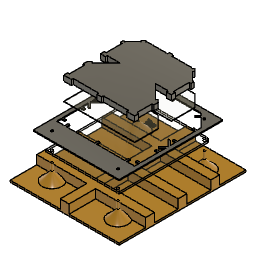
External Panels v20 (Autodesk Fusion 360 design; units mm, degrees)
Autodesk Fusion 360 part; units mm, degrees
note: some values were not read from the file. Chosen so that the rebuilt part matches the saved one: which bodies a step acts on; the layout of a text.
sketch "PCB" plane through (0, 0, 0) normal (0, 0, 1) x (1, 0, 0) in component "ExPan"
  line L0 (-41.5, 51.5) -> (38, 51.5)
  line L1 (41.5, 48) -> (41.5, -51.5)
  line L2 (41.5, -51.5) -> (-41.5, -51.5)
  line L3 (-41.5, -51.5) -> (-41.5, 51.5)
  line L4 (-41.5, 51.5) -> (41.5, -51.5) construction
  line L5 (41.5, 51.5) -> (-41.5, -51.5) construction
  circle A0 centre (-37.3, 49) radius 1.35
  line L6 (-41.5, 0) -> (41.5, 0) construction
  line L7 (0, 51.5) -> (0, -51.5) construction
  circle A1 centre (37.3, 49) radius 1.35
  circle A2 centre (-37.2, -48.5) radius 1.35
  circle A3 centre (37.2, -48.5) radius 1.35
  line L8 (38.907, 51.5) -> (38, 51.5) construction
  arc A4 (41.5, 48) -> (38, 51.5) centre (38, 48) ccw
  dimension "d14" = 83
  dimension "d15" = 103
  dimension "d16" = 2.7
  dimension "d18" = 4.2
  dimension "d19" = 2.5
  dimension "d24" = 2.7
  dimension "d25" = 4.3
  dimension "d26" = 3
  dimension "d141" = 3.5
  constraint horizontal L0
  constraint perpendicular L0 L1
  constraint parallel L0 L2
  constraint parallel L1 L3
  constraint coincident L4 origin
  constraint coincident L5 origin
  constraint midpoint L3 L6.start
  constraint midpoint L2 L7.end
  constraint symmetric A0 L7 A1
  constraint symmetric L7 A2 A3
  constraint horizontal L8
  constraint coincident L0 L8.start
  constraint coincident L1 L6.end
  constraint coincident L5.start L1
  constraint tangent L8 A4
  constraint tangent L1 A4
  constraint coincident L0 L7.start
  measures "d14" distance of L1 L3
  measures "d15" distance of L0 L2
  measures "d16" diameter of A0
  measures "d18" distance of L3 A0.centre
  measures "d19" distance of L0 A0.centre
  measures "d24" diameter of A2
  measures "d25" distance of L3 A2.centre
  measures "d26" distance of L2 A2.centre
  measures "d141" radius of A4
sketch "Base" plane through (0, 0, 0) normal (0, 0, 1) x (1, 0, 0) in component "ExPan"
  line L0 (61.5, -71.5) -> (-61.5, -71.5)
  line L1 (-61.5, -71.5) -> (-61.5, 71.5)
  line L2 (-61.5, 71.5) -> (61.5, 71.5)
  line L3 (61.5, 71.5) -> (61.5, -71.5)
  line L4 (61.5, -71.5) -> (-61.5, 71.5) construction
  line L5 (-61.5, -71.5) -> (61.5, 71.5) construction
  line L6 (41.5, -51.5) -> (-41.5, -51.5)
  line L7 (41.5, 48) -> (41.5, -51.5)
  circle A0 centre (37.2, -48.5) radius 1.1
  line L8 (0, 51.5) -> (0, -51.5) construction
  circle A1 centre (-37.2, -48.5) radius 1.1
  line L9 (-41.5, 0) -> (41.5, 0) construction
  circle A2 centre (37.3, 49) radius 1.1
  line L10 (-41.5, 51.5) -> (38, 51.5)
  circle A3 centre (-37.3, 49) radius 1.1
  line L11 (-61.5, -31.5) -> (61.5, -31.5)
  line L12 (61.5, -31.5) -> (61.5, -41.5)
  line L13 (61.5, -41.5) -> (-61.5, -41.5)
  line L14 (-61.5, -41.5) -> (-61.5, -31.5)
  line L15 (-61.5, 42) -> (61.5, 42)
  line L16 (61.5, 42) -> (61.5, 32)
  line L17 (61.5, 32) -> (-61.5, 32)
  line L18 (-61.5, 32) -> (-61.5, 42)
  line L19 (-5, 71.5) -> (5, 71.5)
  line L20 (5, 71.5) -> (5, -71.5)
  line L21 (5, -71.5) -> (-5, -71.5)
  line L22 (-5, -71.5) -> (-5, 71.5)
  line L23 (-61.5, 5) -> (61.5, 5)
  line L24 (61.5, 5) -> (61.5, -5)
  line L25 (61.5, -5) -> (-61.5, -5)
  line L26 (-61.5, -5) -> (-61.5, 5)
  line L27 (-42.5017, 60.3845) -> (-15.0062, 60.3658) construction
  line L28 (-15.0062, 60.3658) -> (-15.0027, 65.4577) construction
  line L29 (-15.0027, 65.4577) -> (-42.4983, 65.4765) construction
  line L30 (-42.4983, 65.4765) -> (-42.5017, 60.3845) construction
  point P0 (-37.3, 49)
  point P1 (37.3, 49)
  dimension "d35" = 20
  dimension "d36" = 20
  dimension "d37" = 2.2
  dimension "d38" = 3
  dimension "d39" = 4.3
  dimension "d40" = 2.2
  dimension "d41" = 4.2
  dimension "d42" = 2.5
  dimension "d119" = 10
  dimension "d120" = 7
  dimension "d121" = 7
  dimension "d122" = 10
  dimension "d123" = 10
  dimension "d129" = 10
  dimension "d130" = 5
  dimension "d131" = 5
  dimension "d134" = 5
  dimension "d139" = 19
  text T0 "Top" font "Arial" height 5 align left top in box 27.4956 x 5.0919 at (-42.5017, 60.3845) x (1, -0.000682) y (0.000682, 1) spacing 1 kerned
  constraint horizontal L0
  constraint perpendicular L0 L1
  constraint parallel L0 L2
  constraint parallel L1 L3
  constraint coincident L4 origin
  constraint coincident L5 origin
  constraint symmetric A0 L8 A1
  constraint symmetric L8 A2 A3
  constraint horizontal L11
  constraint vertical L12
  constraint horizontal L13
  constraint vertical L14
  constraint coincident L1 L11.start
  constraint horizontal L15
  constraint vertical L16
  constraint horizontal L17
  constraint vertical L18
  constraint coincident L3 L16.end
  constraint coincident L1 L15.start
  constraint horizontal L19
  constraint vertical L20
  constraint horizontal L21
  constraint vertical L22
  constraint coincident L0 L20.end
  constraint coincident L2 L19.start
  constraint horizontal L23
  constraint vertical L24
  constraint horizontal L25
  constraint vertical L26
  constraint coincident L3 L24.end
  constraint coincident L1 L23.start
  measures "d35" distance of L0 L6
  measures "d36" distance of L3 L7
  measures "d37" diameter of A0
  measures "d38" distance of L6 A0.centre
  measures "d39" distance of L7 A0.centre
  measures "d40" diameter of A2
  measures "d41" distance of L7 P1
  measures "d42" distance of P1 L10
  measures "d119" distance of L11.start L13.end
  measures "d120" distance of A1.centre L13
  measures "d121" distance of P0 L15
  measures "d122" distance of L15 L17
  measures "d123" distance of L20 L22
  measures "d129" distance of L23 L25
  measures "d130" distance of origin L23
  measures "d131" distance of origin L22
sketch "SC" plane through (0, 0, 0) normal (0, 0, 1) x (1, 0, 0) in component "ExPan"
  line L0 (-40, 9) -> (40, 9)
  line L1 (40, 9) -> (40, 35.5)
  line L2 (26.5, 49) -> (-26.5, 49)
  line L3 (-40, 35.5) -> (-40, 9)
  line L4 (-41.5, -51.5) -> (-41.5, 51.5)
  line L5 (-41.5, 51.5) -> (38, 51.5)
  line L6 (-40, 35.5) -> (-26.5, 49)
  line L7 (0, 51.5) -> (0, -51.5)
  line L8 (40, 35.5) -> (26.5, 49)
  line L9 (-40, -32.5) -> (40, -32.5)
  line L10 (40, -32.5) -> (40, -6)
  line L11 (26.5, 7.5) -> (-26.5, 7.5)
  line L12 (-40, -6) -> (-26.5, 7.5)
  line L13 (-40, -6) -> (-40, -32.5)
  line L14 (40, -6) -> (26.5, 7.5)
  dimension "d43" = 80
  dimension "d45" = 1.5
  dimension "d47" = 2.5
  dimension "d48" = 13.5
  dimension "d49" = 13.5
  dimension "d190" = 40
  dimension "d191" = 80
  dimension "d192" = 13.5
  dimension "d193" = 13.5
  dimension "d194" = 40
  dimension "d195" = 1.5
  dimension "d196" = 1.5
  constraint vertical L1
  constraint horizontal L2
  constraint vertical L3
  constraint coincident L3.start L6.start
  constraint coincident L2.end L6.end
  constraint symmetric L3.start L7 L1.end
  constraint symmetric L2.end L7 L2.start
  constraint vertical L10
  constraint horizontal L11
  constraint vertical L13
  constraint coincident L12.start L13.start
  constraint coincident L11.end L12.end
  constraint symmetric L7 L11.end L11.start
  constraint symmetric L7 L12.start L10.end
  measures "d43" distance of L0.start L0.end
  measures "d45" distance of L3 L4
  measures "d47" distance of L2 L5
  measures "d48" distance of L2 L3.start
  measures "d49" distance of L3 L2.end
  measures "d190" distance of L0 L2
  measures "d191" distance of L9.start L9.end
  measures "d192" distance of L12.start L11
  measures "d193" distance of L11.end L13
  measures "d194" distance of L9 L11
  measures "d195" distance of L0 L11
  measures "d196" distance of L4 L13
sketch "Mask" plane through (0, 0, 0) normal (0, 0, 1) x (1, 0, 0) in component "ExPan"
  line L0 (-45, 58.5) -> (48.5, 58.5)
  line L1 (48.5, 58.5) -> (48.5, -58.5)
  line L2 (48.5, -58.5) -> (-48.5, -58.5)
  line L3 (-48.5, -58.5) -> (-48.5, 58.5)
  line L4 (-41.5, -51.5) -> (-41.5, 51.5)
  line L5 (41.5, -51.5) -> (-41.5, -51.5)
  circle A0 centre (-37.2, -48.5) radius 1.35
  circle A1 centre (-37.3, 49) radius 1.35
  line L6 (-48.5, 58.5) -> (-45, 58.5)
  line L7 (44, -36.5) -> (44, 38.5711)
  line L8 (44, 38.5711) -> (29.5711, 53)
  line L9 (29.5711, 53) -> (-29.5711, 53)
  line L10 (-44, 38.5711) -> (-44, -36.5)
  line L11 (17.1694, 53) -> (17.1971, 53)
  line L12 (17.1971, 50.5) -> (17.1694, 50.5)
  line L13 (-41.5, 51.5) -> (38, 51.5)
  line L14 (-44, -36.5) -> (44, -36.5)
  line L15 (-29.5711, 53) -> (-44, 38.5711)
  line L16 (-40, 35.5) -> (-26.5, 49)
  line L17 (40, 35.5) -> (26.5, 49)
  line L18 (-40, -32.5) -> (40, -32.5)
  line L19 (0, 51.5) -> (0, -51.5)
  circle A2 centre (37.2, -48.5) radius 1.35
  circle A3 centre (37.3, 49) radius 1.35
  line L20 (-40.1, -6) -> (-40.1, -35)
  line L21 (-40, -6) -> (-40, -32.5)
  line L22 (-44, -31.4682) -> (-40.1, -31.4682)
  line L23 (-44, -29.4682) -> (-40.1, -29.4682)
  line L24 (40.1, -6) -> (40.1, -35)
  line L25 (-26.5404, 7.601) -> (-41.5185, -7.3771)
  line L26 (-26.5404, 7.601) -> (-5.482, 7.601) construction
  line L27 (-40, -6) -> (-26.5, 7.5)
  line L28 (-39.6133, -5.4719) -> (-44, -1.0852)
  line L29 (-39.6133, -5.4719) -> (-31.8598, -5.4719) construction
  line L30 (-38.1991, -4.0577) -> (-44, 1.7432)
  line L31 (-38.1991, -4.0577) -> (-31.6288, -4.0577) construction
  line L32 (-44, -7.8862) -> (-40.1, -7.8862)
  line L33 (-44, -9.8862) -> (-40.1, -9.8862)
  line L34 (-41, -32.6) -> (42, -32.6)
  line L35 (-34.94, -36.5) -> (-34.94, -32.6)
  line L36 (-32.94, -36.5) -> (-32.94, -32.6)
  line L37 (-1, -36.5) -> (-1, -32.6)
  line L38 (1, -36.5) -> (1, -32.6)
  line L39 (34.94, -36.5) -> (34.94, -32.6)
  line L40 (32.94, -36.5) -> (32.94, -32.6)
  line L41 (44, -31.4682) -> (40.1, -31.4682)
  line L42 (44, -29.4682) -> (40.1, -29.4682)
  line L43 (44, -9.8862) -> (40.1, -9.8862)
  line L44 (44, -7.8862) -> (40.1, -7.8862)
  line L45 (38.1991, -4.0577) -> (44, 1.7432)
  line L46 (39.6133, -5.4719) -> (44, -1.0852)
  line L47 (26.5404, 7.601) -> (41.5185, -7.3771)
  line L48 (26.5, 49) -> (-26.5, 49)
  line L49 (-26.1265, 49.15) -> (28.8735, 49.15)
  line L50 (-40.1, 8) -> (-40.1, 37)
  line L51 (-40, 35.5) -> (-40, 9)
  line L52 (-40.0495, 35.5919) -> (-25.6143, 50.0271)
  line L53 (-44, 34.0706) -> (-40.1, 34.0706)
  line L54 (-44, 32.0706) -> (-40.1, 32.0706)
  line L55 (-40.1, 11.9824) -> (-44, 11.9824)
  line L56 (-44, 9.9824) -> (-40.1, 9.9824)
  line L57 (-1, 53) -> (-1, 49.15)
  line L58 (-33.213, 49.358) -> (-29.7482, 45.8932)
  line L59 (-31.7988, 50.7723) -> (-28.334, 47.3074)
  line L60 (-41, 8.9) -> (42.4266, 8.9)
  line L61 (-40, 9) -> (40, 9)
  line L62 (39.1562, 8.9) -> (44, 4.0562)
  line L63 (39.1562, 8.9) -> (45.9442, 8.9) construction
  line L64 (36.3278, 8.9) -> (44.4159, 0.8118)
  line L65 (36.3278, 8.9) -> (47.7041, 8.9) construction
  line L66 (-36.3278, 8.9) -> (-44.4159, 0.8118)
  line L67 (-39.1562, 8.9) -> (-44, 4.0562)
  line L68 (33.213, 49.358) -> (29.7482, 45.8932)
  line L69 (31.7988, 50.7723) -> (28.334, 47.3074)
  line L70 (1, 53) -> (1, 49.15)
  line L71 (44, 34.0706) -> (40.1, 34.0706)
  line L72 (44, 32.0706) -> (40.1, 32.0706)
  line L73 (40.1, 11.9824) -> (44, 11.9824)
  line L74 (44, 9.9824) -> (40.1, 9.9824)
  line L75 (40.0495, 35.5919) -> (25.6143, 50.0271)
  line L76 (40.1, 8) -> (40.1, 37)
  dimension "d55" = 117
  dimension "d56" = 97
  dimension "d58" = 7
  dimension "d59" = 7
  dimension "d99" = 2.7
  dimension "d100" = 11.3
  dimension "d101" = 10
  dimension "d102" = 2.7
  dimension "d103" = 11.2
  dimension "d104" = 9.5
  dimension "d182" = 4.5
  dimension "d183" = 4.5
  dimension "d185" = 5
  dimension "d198" = 5
  dimension "d199" = 4
  dimension "d200" = 0.1
  dimension "d201" = 2
  dimension "d202" = 135
  dimension "d203" = 0.1
  dimension "d204" = 135
  dimension "d205" = 135
  dimension "d206" = 2
  dimension "d207" = 2
  dimension "d208" = 0.1
  dimension "d209" = 2
  dimension "d210" = 1
  dimension "d211" = 4
  dimension "d212" = 0.15
  dimension "d213" = 0.1
  dimension "d214" = 2
  dimension "d215" = 2
  dimension "d216" = 1
  dimension "d217" = 0.1
  dimension "d218" = 2
  dimension "d219" = 0.1
  dimension "d220" = 45
  dimension "d221" = 45
  dimension "d222" = 2
  constraint horizontal L0
  constraint vertical L1
  constraint horizontal L2
  constraint vertical L3
  constraint horizontal L6
  constraint vertical L10
  constraint horizontal L11
  constraint horizontal L12
  constraint coincident L9 L11.start
  constraint symmetric A0 L19 A2
  constraint symmetric A1 L19 A3
  constraint parallel L4 L20
  constraint coincident L10 L22.start
  constraint coincident L20 L22.end
  constraint perpendicular L20 L22
  constraint coincident L10 L23.start
  constraint coincident L20 L23.end
  constraint perpendicular L20 L23
  constraint symmetric L19 L20.start L24.start
  constraint symmetric L19 L20.end L24.end
  constraint horizontal L26
  constraint horizontal L29
  constraint coincident L25 L28.start
  constraint coincident L10 L28.end
  constraint horizontal L31
  constraint coincident L25 L30.start
  constraint coincident L10 L30.end
  constraint coincident L10 L32.start
  constraint coincident L20 L32.end
  constraint perpendicular L20 L32
  constraint coincident L10 L33.start
  constraint coincident L20 L33.end
  constraint perpendicular L20 L33
  constraint perpendicular L7 L34
  constraint coincident L14 L35.start
  constraint coincident L34 L35.end
  constraint perpendicular L34 L35
  constraint coincident L14 L36.start
  constraint coincident L34 L36.end
  constraint perpendicular L18 L36
  constraint coincident L14 L37.start
  constraint coincident L34 L37.end
  constraint perpendicular L34 L37
  constraint symmetric L19 L22.start L41.start
  constraint symmetric L19 L22.end L41.end
  constraint symmetric L19 L23.start L42.start
  constraint symmetric L19 L23.end L42.end
  constraint symmetric L19 L25.start L47.start
  constraint symmetric L19 L25.end L47.end
  constraint symmetric L19 L28.start L46.start
  constraint symmetric L19 L28.end L46.end
  constraint symmetric L19 L30.start L45.start
  constraint symmetric L19 L30.end L45.end
  constraint symmetric L19 L32.start L44.start
  constraint symmetric L19 L32.end L44.end
  constraint symmetric L19 L33.start L43.start
  constraint symmetric L19 L33.end L43.end
  constraint symmetric L19 L35.start L39.start
  constraint symmetric L19 L35.end L39.end
  constraint symmetric L19 L36.start L40.start
  constraint symmetric L19 L36.end L40.end
  constraint symmetric L19 L37.start L38.start
  constraint symmetric L19 L37.end L38.end
  constraint parallel L48 L49
  constraint parallel L4 L50
  constraint parallel L16 L52
  constraint coincident L10 L53.start
  constraint coincident L50 L53.end
  constraint perpendicular L50 L53
  constraint coincident L10 L54.start
  constraint coincident L50 L54.end
  constraint perpendicular L50 L54
  constraint coincident L50 L55.start
  constraint coincident L10 L55.end
  constraint perpendicular L10 L55
  constraint coincident L10 L56.start
  constraint coincident L50 L56.end
  constraint perpendicular L50 L56
  constraint coincident L9 L57.start
  constraint coincident L49 L57.end
  constraint perpendicular L49 L57
  constraint coincident L15 L58.start
  constraint coincident L52 L58.end
  constraint perpendicular L52 L58
  constraint coincident L15 L59.start
  constraint coincident L52 L59.end
  constraint perpendicular L52 L59
  constraint perpendicular L51 L60
  constraint horizontal L63
  constraint coincident L60 L62.start
  constraint coincident L7 L62.end
  constraint horizontal L65
  constraint coincident L60 L64.start
  constraint symmetric L19 L53.start L71.start
  constraint symmetric L19 L53.end L71.end
  constraint symmetric L19 L54.start L72.start
  constraint symmetric L19 L54.end L72.end
  constraint symmetric L19 L55.start L73.start
  constraint symmetric L19 L55.end L73.end
  constraint symmetric L19 L56.start L74.start
  constraint symmetric L19 L56.end L74.end
  constraint symmetric L19 L57.start L70.start
  constraint symmetric L19 L57.end L70.end
  constraint symmetric L19 L58.start L68.start
  constraint symmetric L19 L58.end L68.end
  constraint symmetric L19 L59.start L69.start
  constraint symmetric L19 L59.end L69.end
  constraint symmetric L19 L62.start L67.start
  constraint symmetric L19 L62.end L67.end
  constraint symmetric L19 L64.start L66.start
  constraint symmetric L19 L64.end L66.end
  constraint symmetric L19 L50.start L76.start
  constraint symmetric L19 L50.end L76.end
  constraint symmetric L19 L52.start L75.start
  constraint symmetric L19 L52.end L75.end
  measures "d55" distance of L0 L2
  measures "d56" distance of L1 L3
  measures "d58" distance of L3 L4
  measures "d59" distance of L2 L5
  measures "d99" diameter of A0
  measures "d100" distance of L3 A0.centre
  measures "d101" distance of L2 A0.centre
  measures "d102" diameter of A1
  measures "d103" distance of L3 A1.centre
  measures "d104" distance of L0 A1.centre
  measures "d182" distance of L3 L10
  measures "d183" distance of L1 L7
  measures "d185" distance of L15 L16
  measures "d198" distance of L8 L17
  measures "d199" distance of L14 L18
  measures "d200" distance of L20 L21
  measures "d201" distance of L22 L23
  measures "d202" angle of L25 L26
  measures "d203" distance of L25 L27
  measures "d204" angle of L28 L29
  measures "d205" angle of L30 L31
  measures "d206" distance of L28 L30
  measures "d207" distance of L32 L33
  measures "d208" distance of L18 L34
  measures "d209" distance of L35 L36
  measures "d210" distance of L19 L37
  measures "d211" distance of L9 L48
  measures "d212" distance of L48 L49
  measures "d213" distance of L50 L51
  measures "d214" distance of L53 L54
  measures "d215" distance of L55 L56
  measures "d216" distance of L19.start L57
  measures "d217" distance of L16 L52
  measures "d218" distance of L58 L59
  measures "d219" distance of L60 L61
  measures "d220" angle of L62 L63
  measures "d221" angle of L64 L65
  measures "d222" distance of L62 L64
extrude "Extrude11" add sketch "Base" along normal blind 20 contours A0 | A1 | A2 | A3 makes body 1 at (-36.1014, -48.5548, 13.3333) makes body 2 at (38.3986, 48.9452, 13.3333) makes body 3 at (38.2986, -48.5548, 13.3333) makes body 4 at (-36.2014, 48.9452, 13.3333) in component "ExPan"
extrude "Extrude12" add sketch "Base" along normal blind 2 separate body makes body 5 in component "ExPan"
combine "Combine3" operation add target body 5 tool bodies 1 4 2 3 in component "ExPan"
fillet "Fillet1" radius 10 tangency weight 0.1 1 edges at (-38.2256, -48.1022, 2) on bodies 5 in component "ExPan"
fillet "Fillet2" radius 10 tangency weight 0.1 1 edges at (-38.3256, 49.3978, 2) on bodies 5 in component "ExPan"
fillet "Fillet3" radius 1 1 edges at (-61.5, 71.5, 1) on bodies 5 in component "ExPan"
fillet "Fillet4" radius 10 tangency weight 0.1 1 edges at (36.2744, 49.3978, 2) on bodies 5 in component "ExPan"
fillet "Fillet5" radius 10 tangency weight 0.1 1 edges at (36.1744, -48.1022, 2) on bodies 5 in component "ExPan"
extrude "Extrude19" add sketch "Base" along normal blind 12 separate body contours L0 L6 L20 L21 L22 | L3 L7 L11 L12 L13 | L6 L13 L20 L22 | L7 L11 L13 L20 | L11 L13 L20 L22 | L3 L7 L23 L24 L25 | L1 L11 L13 L14 L22 | L11 L20 L22 L25 | L7 L20 L23 L25 | L20 L22 L23 L25 | L3 L7 L15 L16 L17 | L1 L22 L23 L25 L26 | L17 L20 L22 L23 | L7 L15 L17 L20 | L15 L17 L20 L22 | L1 L15 L17 L18 L22 | L10 L15 L20 L22 | L2 L10 L19 L20 L22 makes body 6 in component "ExPan"
extrude "Extrude20" add sketch "Base" along normal blind 3 separate body text T0 makes body 7 at (-34.8275, 60.7532, 1) makes body 8 at (-38.7106, 62.5352, 0) makes body 9 at (-40.8533, 61.9453, 1) in component "ExPan"
combine "Combine4" operation add target body 5 tool bodies 6 in component "ExPan"
combine "Combine5" operation add target body 5 tool bodies 8 7 9 in component "ExPan"
sketch "Press" plane through (0, 0, 0) normal (0, 0, 1) x (1, 0, 0) in component "ExPan"
  line L0 (-38, -6.8284) -> (-20.1716, 11)
  line L1 (-39.0929, -6.5071) -> (-13.7265, -6.5071) construction
  line L2 (-40, -6) -> (-26.5, 7.5)
  line L3 (-38, -30.5) -> (-38, -6.8284)
  line L4 (-40, -6) -> (-40, -32.5)
  line L5 (-38, -30.5) -> (38, -30.5)
  line L6 (-40, -32.5) -> (40, -32.5)
  line L7 (0, 51.5) -> (0, -51.5)
  line L8 (38, -30.5) -> (38, -6.8284)
  line L9 (-38, 11) -> (-20.1716, 11)
  line L10 (-40, 9) -> (40, 9)
  line L11 (-38, 34.6716) -> (-38, 11)
  line L12 (-40, 35.5) -> (-40, 9)
  line L13 (-38, 34.6716) -> (-25.6716, 47)
  line L14 (-38, 34.6716) -> (-10.6154, 34.6716) construction
  line L15 (-25.6716, 47) -> (25.6716, 47)
  line L16 (-40, 35.5) -> (-26.5, 49)
  line L17 (26.5, 49) -> (-26.5, 49)
  line L18 (38, 11) -> (20.1716, 11)
  line L19 (-40, 9) -> (40, 9)
  line L20 (25.6716, 47) -> (38, 34.6716)
  line L21 (25.6716, 47) -> (42.9596, 47) construction
  line L22 (40, 35.5) -> (26.5, 49)
  line L23 (38, 34.6716) -> (38, 11)
  line L24 (40, 9) -> (40, 35.5)
  line L25 (20.1716, 11) -> (38, -6.8284)
  line L26 (-30.3408, 45.1592) -> (-28.9266, 43.745)
  line L27 (-27.6755, 47.8245) -> (-26.2613, 46.4103)
  line L28 (-30.3408, 45.1592) -> (-27.6755, 47.8245)
  line L29 (27.6755, 47.8245) -> (30.3408, 45.1592)
  line L30 (-38, -10.8515) -> (-40, -10.8515)
  line L31 (-40, -6) -> (-37.2197, -3.2197)
  line L32 (-35.8055, -4.6339) -> (-37.2197, -3.2197)
  line L33 (-31.1666, -32.5) -> (-31.1666, -30.5)
  line L34 (-6.0474, 47) -> (-2.2729, 47)
  line L35 (-2.2729, 47) -> (-2.2729, 49)
  line L36 (-38, 34.5836) -> (-40, 34.5836)
  line L37 (-38, 31.3042) -> (-40, 31.3042)
  line L38 (-40, 34.5836) -> (-40, 31.3042)
  line L39 (-40, -27.9459) -> (-38, -27.9459)
  line L40 (34.3688, 11) -> (34.3688, 9)
  line L41 (38, 13.4329) -> (40, 13.4329)
  line L42 (-2.6389, -30.5) -> (-2.6389, -32.5)
  line L43 (2.6389, -30.5) -> (2.6389, -32.5)
  line L44 (40, -27.9459) -> (38, -27.9459)
  line L45 (31.1666, -32.5) -> (31.1666, -30.5)
  line L46 (38, -10.8515) -> (40, -10.8515)
  line L47 (35.8055, -4.6339) -> (37.2197, -3.2197)
  line L48 (38, 34.5836) -> (40, 34.5836)
  line L49 (40, 34.5836) -> (40, 31.3042)
  line L50 (38, 31.3042) -> (40, 31.3042)
  line L51 (27.6755, 47.8245) -> (26.2613, 46.4103)
  line L52 (30.3408, 45.1592) -> (28.9266, 43.745)
  line L53 (30.3408, 45.1592) -> (27.6755, 47.8245)
  line L54 (2.2729, 47) -> (2.2729, 49)
  line L55 (-2.2729, 49) -> (2.2729, 49)
  line L56 (-40, -27.9459) -> (-40, -32.5)
  line L57 (-2.6389, -32.5) -> (2.6389, -32.5)
  line L58 (31.1666, -32.5) -> (40, -32.5)
  line L59 (40, -27.9459) -> (40, -32.5)
  line L60 (34.3688, 9) -> (40, 9)
  line L61 (40, 13.4329) -> (40, 9)
  line L62 (-38, 13.4329) -> (-40, 13.4329)
  line L63 (-34.3688, 11) -> (-34.3688, 9)
  line L64 (-40, 13.4329) -> (-40, 9)
  line L65 (-34.3688, 9) -> (-40, 9)
  line L66 (-40, -6) -> (-40, -10.8515)
  line L67 (40, -6) -> (40, -10.8515)
  line L68 (40, -6) -> (37.2197, -3.2197)
  line L69 (-20.1716, 11) -> (20.1716, 11)
  line L70 (26.5, 7.5) -> (-26.5, 7.5)
  line L71 (-25.6716, 5.5) -> (25.6716, 5.5)
  dimension "d223" = 45
  dimension "d224" = 2
  dimension "d225" = 2
  dimension "d226" = 2
  dimension "d227" = 2
  dimension "d228" = 2
  dimension "d229" = 45
  dimension "d230" = 2
  dimension "d231" = 2
  dimension "d232" = 2
  dimension "d233" = 45
  dimension "d234" = 2
  dimension "d235" = 2
  constraint horizontal L1
  constraint perpendicular L1 L3
  constraint perpendicular L3 L5
  constraint symmetric L3.start L7 L5.end
  constraint symmetric L0.start L7 L8.end
  constraint horizontal L9
  constraint perpendicular L10 L11
  constraint horizontal L14
  constraint parallel L14 L15
  constraint horizontal L18
  constraint horizontal L21
  constraint vertical L23
  constraint coincident L16 L26.start
  constraint coincident L13 L26.end
  constraint perpendicular L13 L26
  constraint coincident L16 L27.start
  constraint coincident L13 L27.end
  constraint perpendicular L13 L27
  constraint perpendicular L27 L28
  constraint symmetric L7 L26.start L29.end
  constraint symmetric L7 L27.start L29.start
  constraint coincident L3 L30.start
  constraint coincident L4 L30.end
  constraint perpendicular L4 L30
  constraint coincident L2.start L4.start
  constraint coincident L2 L31.end
  constraint parallel L2 L31
  constraint coincident L0 L32.start
  constraint perpendicular L2 L32
  constraint coincident L6 L33.start
  constraint coincident L5 L33.end
  constraint perpendicular L5 L33
  constraint horizontal L34
  constraint vertical L35
  constraint coincident L17 L35.end
  constraint coincident L15 L34.start
  constraint coincident L11 L36.start
  constraint coincident L12 L36.end
  constraint perpendicular L12 L36
  constraint coincident L11 L37.start
  constraint coincident L12 L37.end
  constraint perpendicular L12 L37
  constraint perpendicular L37 L38
  constraint coincident L4 L39.start
  constraint perpendicular L4 L39
  constraint coincident L18 L40.start
  constraint perpendicular L18 L40
  constraint coincident L23 L41.start
  constraint coincident L24 L41.end
  constraint perpendicular L24 L41
  constraint coincident L5 L42.start
  constraint coincident L6 L42.end
  constraint perpendicular L6 L42
  constraint symmetric L7 L26.end L52.end
  constraint symmetric L7 L27.end L51.end
  constraint symmetric L7 L30.start L46.start
  constraint symmetric L7 L30.end L46.end
  constraint symmetric L7 L31.end L47.end
  constraint symmetric L7 L32.start L47.start
  constraint symmetric L7 L33.start L45.start
  constraint symmetric L7 L33.end L45.end
  constraint symmetric L7 L34.end L54.start
  constraint symmetric L7 L35.end L54.end
  constraint symmetric L7 L36.start L48.start
  constraint symmetric L7 L36.end L48.end
  constraint symmetric L7 L37.start L50.start
  constraint symmetric L7 L37.end L49.end
  constraint symmetric L7 L39.start L44.start
  constraint symmetric L7 L39.end L44.end
  constraint symmetric L7 L42.start L43.start
  constraint symmetric L7 L42.end L43.end
  constraint coincident L4.end L6.start
  constraint coincident L6.end L58.end
  constraint coincident L10.end L19.end
  constraint perpendicular L10 L61
  constraint symmetric L7 L40.start L63.start
  constraint symmetric L7 L40.end L63.end
  constraint symmetric L7 L41.start L62.start
  constraint symmetric L7 L41.end L62.end
  constraint symmetric L7 L10.end L10.start
  constraint symmetric L7 L2.start L67.start
  constraint parallel L18 L69
  constraint coincident L0 L71.start
  constraint coincident L25 L71.end
  measures "d223" angle of L0 L1
  measures "d224" distance of L0 L2
  measures "d225" distance of L3 L4
  measures "d226" distance of L5 L6
  measures "d227" distance of L9 L10
  measures "d228" distance of L11 L12
  measures "d229" angle of L13 L14
  measures "d230" distance of L13 L16
  measures "d231" distance of L15 L17
  measures "d232" distance of L18 L19
  measures "d233" angle of L20 L21
  measures "d234" distance of L20 L22
  measures "d235" distance of L23 L24
extrude "Extrude22" add sketch "SC" along normal blind 0.4 separate body contours L0 L2 L3 L6 L7 | L0 L1 L2 L7 L8 makes body 10 in component "ExPan"
extrude "Extrude25" add sketch "Mask" along normal blind 1 separate body contours L0 L1 L2 L3 L6 | L4 L5 L14 L19 | L4 L10 L22 L23 | L4 L20 L22 L23 | L14 L34 L35 L36 | L14 L19 L34 L38 | L14 L19 L34 L37 | L4 L10 L32 L33 | L4 L20 L32 L33 | L14 L34 L39 L40 | L4 L60 L66 L67 | L7 L45 L60 L62 L64 | L4 L10 L28 L30 L66 | L4 L25 L28 L30 | L7 L24 L41 L42 | L4 L10 L30 L66 L67 | L7 L45 L46 L47 L64 | L7 L45 L64 | L10 L30 L66 | L13 L19 L49 L57 | L13 L19 L49 L70 | L7 L24 L43 L44 | L9 L13 L57 L70 | L4 L50 L55 L56 | L4 L10 L55 L56 | L7 L73 L74 L76 | L4 L13 L15 | L8 L68 L69 L75 | L4 L50 L53 L54 | L4 L10 L53 L54 | L7 L71 L72 L76 | L15 L52 L58 L59 makes body 11 in component "ExPan"
extrude "Extrude26" add sketch "Press" along normal blind 6 separate body contours L0 L2 L3 L4 L30 L31 L32 L66 | L0 L3 L5 L7 L71 | L0 L7 L70 L71 | L3 L4 L5 L6 L33 L39 L56 | L0 L7 L10 L19 L70 | L5 L7 L8 L25 L71 | L7 L25 L70 L71 | L0 L7 L10 L19 L69 | L7 L10 L19 L25 L70 | L5 L6 L7 L42 L57 | L5 L6 L7 L43 L57 | L7 L9 L11 L13 L15 L34 L69 | L9 L10 L11 L12 L19 L62 L63 L64 L65 | L7 L10 L19 L25 L69 | L8 L25 L46 L47 L67 L68 | L7 L15 L18 L20 L23 L69 | L5 L6 L8 L44 L45 L58 L59 | L7 L15 L17 L35 L55 | L7 L15 L17 L54 L55 | L10 L18 L19 L23 L24 L40 L41 L60 L61 | L11 L12 L36 L37 L38 | L20 L22 L29 L51 L52 L53 | L23 L24 L48 L49 L50 | L13 L16 L26 L27 L28 makes body 12 in component "ExPan"
extrude "Extrude28" cut sketch "Press" along normal blind 3 contours L0 L7 L70 L71 | L0 L7 L10 L19 L70 | L7 L25 L70 L71 | L0 L7 L10 L19 L69 | L7 L10 L19 L25 L70 | L7 L10 L19 L25 L69 bodies 12 in component "ExPan"
extrude "Extrude29" add sketch "PCB" along normal blind 2 separate body makes body 13 in component "ExPan"
extrude "Extrude30" add sketch "SC" along normal blind 0.4 separate body contours L7 L9 L10 L11 L14 | L7 L9 L11 L12 L13 makes body 14 in component "ExPan"
sketch "grid" plane through (0, 0, 0) normal (0, 0, 1) x (1, 0, 0) in component "ExPan"
  line L0 (-40, -6) -> (-40, -32.5)
  line L1 (-40, -6) -> (-26.5, 7.5)
  line L2 (-40, -32.5) -> (40, -32.5)
  line L3 (0, 51.5) -> (0, -51.5)
  line L4 (-36, -25.05) -> (36, -25.05)
  line L5 (-36, -24.65) -> (36, -24.65)
  line L6 (-23.8787, 5.8787) -> (2.5511, 5.8787) construction
  line L7 (23.7431, 4.6) -> (36, -7.6569)
  line L8 (-40, -6) -> (-26.5, 7.5)
  line L9 (-23.7431, 4.6) -> (23.7431, 4.6)
  line L10 (-36, -7.6569) -> (-36, -29.6)
  line L11 (36, -7.6569) -> (36, -29.6)
  line L12 (-36, -29.6) -> (36, -29.6)
  line L13 (-23.7431, 4.6) -> (-36, -7.6569)
  line L14 (48.5, 58.5) -> (48.5, -58.5)
  line L15 (-53.5, 63.5) -> (53.5, 63.5)
  line L16 (-53.5, -63.5) -> (-53.5, 63.5)
  circle A0 centre (-37.2, -48.5) radius 1.35
  circle A1 centre (-37.3, 49) radius 1.35
  circle A2 centre (37.3, 49) radius 1.35
  circle A3 centre (37.2, -48.5) radius 1.35
  line L17 (-36, -20.1) -> (36, -20.1)
  line L18 (-36, -19.7) -> (36, -19.7)
  line L19 (-36, -14.75) -> (36, -14.75)
  line L20 (-36, -15.15) -> (36, -15.15)
  line L21 (-36, -9.8) -> (36, -9.8)
  line L22 (-36, -10.2) -> (36, -10.2)
  line L23 (-33.5931, -5.25) -> (33.5931, -5.25)
  line L24 (-33.1931, -4.85) -> (33.1931, -4.85)
  line L25 (-28.6431, -0.3) -> (28.6431, -0.3)
  line L26 (-28.2431, 0.1) -> (28.2431, 0.1)
  line L27 (26.5, 7.5) -> (-26.5, 7.5)
  line L28 (40, -32.5) -> (40, -6)
  line L29 (-40, -6) -> (-40, -32.5)
  line L30 (40, -6) -> (26.5, 7.5)
  line L31 (-36, 11.9) -> (36, 11.9)
  line L32 (-36, 33.8431) -> (-36, 11.9)
  line L33 (-36, 26.35) -> (36, 26.35)
  line L34 (-36, 26.75) -> (36, 26.75)
  line L35 (-36, 21.8) -> (36, 21.8)
  line L36 (-36, 21.4) -> (36, 21.4)
  line L37 (-36, 16.45) -> (36, 16.45)
  line L38 (-36, 16.85) -> (36, 16.85)
  line L39 (-36, 31.7) -> (36, 31.7)
  line L40 (-36, 31.3) -> (36, 31.3)
  line L41 (-33.5931, 36.25) -> (33.5931, 36.25)
  line L42 (-33.1931, 36.65) -> (33.1931, 36.65)
  line L43 (-23.7431, 46.1) -> (-36, 33.8431)
  line L44 (-28.6431, 41.2) -> (28.6431, 41.2)
  line L45 (-28.2431, 41.6) -> (28.2431, 41.6)
  line L46 (-23.7431, 46.1) -> (23.7431, 46.1)
  line L47 (23.7431, 46.1) -> (36, 33.8431)
  line L48 (36, 33.8431) -> (36, 11.9)
  line L49 (-48.5, -58.5) -> (-48.5, 58.5)
  line L50 (-45, 58.5) -> (48.5, 58.5)
  line L51 (-53.5, -63.5) -> (53.5, -63.5)
  line L52 (48.5, -58.5) -> (-48.5, -58.5)
  line L53 (53.5, -63.5) -> (53.5, 63.5)
  dimension "d264" = 135
  dimension "d266" = 4
  dimension "d268" = 2.7
  dimension "d269" = 2.7
  dimension "d270" = 2.7
  dimension "d271" = 2.7
  dimension "d278" = 4.55
  dimension "d280" = 0.4
  dimension "d281" = 2.9
  dimension "d285" = 0.4
  dimension "d286" = 0.4
  dimension "d287" = 0.4
  dimension "d288" = 0.4
  dimension "d291" = 4.55
  dimension "d292" = 4.55
  dimension "d293" = 4.55
  dimension "d294" = 4.55
  dimension "d295" = 4.55
  dimension "d296" = 0.4
  dimension "d297" = 2.9
  dimension "d298" = 4
  dimension "d299" = 4
  dimension "d300" = 4
  dimension "d314" = 4.55
  dimension "d315" = 0.4
  dimension "d316" = 0.4
  dimension "d317" = 0.4
  dimension "d318" = 0.4
  dimension "d319" = 0.4
  dimension "d320" = 4.55
  dimension "d321" = 4.55
  dimension "d322" = 4.55
  dimension "d323" = 4.55
  dimension "d324" = 4.55
  dimension "d325" = 0.4
  dimension "d326" = 5
  dimension "d327" = 5
  dimension "d328" = 5
  dimension "d329" = 5
  constraint horizontal L6
  constraint horizontal L15
  constraint coincident L11 L4.end
  constraint coincident L11 L5.end
  constraint coincident L13 L25.start
  constraint coincident L13 L26.start
  constraint coincident L13 L24.start
  constraint coincident L13 L23.start
  constraint coincident L7 L26.end
  constraint coincident L7 L25.end
  constraint coincident L7 L24.end
  constraint coincident L7 L23.end
  constraint coincident L10 L22.start
  constraint coincident L10 L21.start
  constraint coincident L10 L19.start
  constraint coincident L10 L20.start
  constraint coincident L10 L18.start
  constraint coincident L10 L17.start
  constraint coincident L10 L4.start
  constraint coincident L10 L5.start
  constraint coincident L11 L17.end
  constraint coincident L11 L18.end
  constraint coincident L11 L20.end
  constraint coincident L11 L19.end
  constraint coincident L11 L21.end
  constraint coincident L11 L22.end
  constraint coincident L37.end L48
  constraint coincident L38.end L48
  constraint coincident L44.start L43
  constraint coincident L45.start L43
  constraint coincident L42.start L43
  constraint coincident L41.start L43
  constraint coincident L45.end L47
  constraint coincident L44.end L47
  constraint coincident L42.end L47
  constraint coincident L41.end L47
  constraint coincident L40.start L32
  constraint coincident L39.start L32
  constraint coincident L34.start L32
  constraint coincident L33.start L32
  constraint coincident L35.start L32
  constraint coincident L36.start L32
  constraint coincident L37.start L32
  constraint coincident L38.start L32
  constraint coincident L36.end L48
  constraint coincident L35.end L48
  constraint coincident L33.end L48
  constraint coincident L34.end L48
  constraint coincident L39.end L48
  constraint coincident L40.end L48
  constraint perpendicular L16 L51
  constraint perpendicular L51 L53
  measures "d264" angle of L6 L13
  measures "d266" distance of L8 L13
  measures "d268" diameter of A0
  measures "d269" diameter of A1
  measures "d270" diameter of A2
  measures "d271" diameter of A3
  measures "d278" distance of L4 L12
  measures "d280" distance of L4 L5
  measures "d281" distance of L2 L12
  measures "d285" distance of L17 L18
  measures "d286" distance of L19 L20
  measures "d287" distance of L21 L22
  measures "d288" distance of L23 L24
  measures "d291" distance of L5 L17
  measures "d292" distance of L18 L20
  measures "d293" distance of L19 L22
  measures "d294" distance of L21 L23
  measures "d295" distance of L24 L25
  measures "d296" distance of L25 L26
  measures "d297" distance of L9 L27
  measures "d298" distance of L11 L28
  measures "d299" distance of L10 L29
  measures "d300" distance of L7 L30
  measures "d314" distance of L31 L37
  measures "d315" distance of L37 L38
  measures "d316" distance of L35 L36
  measures "d317" distance of L33 L34
  measures "d318" distance of L39 L40
  measures "d319" distance of L41 L42
  measures "d320" distance of L36 L38
  measures "d321" distance of L33 L35
  measures "d322" distance of L34 L40
  measures "d323" distance of L39 L41
  measures "d324" distance of L42 L44
  measures "d325" distance of L44 L45
  measures "d326" distance of L16 L49
  measures "d327" distance of L15 L50
  measures "d328" distance of L51 L52
  measures "d329" distance of L14 L53
move_body "Move13" bodies 12 to x (1, 0, 0) y (0, 1, 0) z (0, 0, 1) at (0, 0, 150) in component "ExPan"
move_body "Move14" bodies 12 to x (1, 0, 0) y (0, 1, 0) z (0, 0, 1) at (0, 0, -100) in component "ExPan"
move_body "Move15" bodies 12 to x (1, 0, 0) y (0, 1, 0) z (0, 0, 1) at (0, 0, -20) in component "ExPan"
move_body "Move16" bodies 13 to x (1, 0, 0) y (0, 1, 0) z (0, 0, 1) at (0, 0, -20) in component "ExPan"
move_body "Move17" bodies 12 to x (1, 0, 0) y (0, 1, 0) z (0, 0, 1) at (0, 0, -10) in component "ExPan"
move_body "Move18" bodies 13 to x (1, 0, 0) y (0, 1, 0) z (0, 0, 1) at (0, 0, -30) in component "ExPan"
move_body "Move19" bodies 11 to x (1, 0, 0) y (0, 1, 0) z (0, 0, 1) at (0, 0, -15) in component "ExPan"
move_body "Move20" bodies 13 to x (1, 0, 0) y (0, 1, 0) z (0, 0, 1) at (0, 0, 10) in component "ExPan"
move_body "Move21" bodies 5 to x (1, 0, 0) y (0, 1, 0) z (0, 0, 1) at (0, 0, -70) in component "ExPan"
move_body "Move22" bodies 13 to x (1, 0, 0) y (0, 1, 0) z (0, 0, 1) at (0, 0, 5) in component "ExPan"
move_body "Move23" bodies 13 to x (1, 0, 0) y (0, 1, 0) z (0, 0, 1) at (0, 0, -5) in component "ExPan"
move_body "Move24" bodies 11 to x (1, 0, 0) y (0, 1, 0) z (0, 0, 1) at (0, 0, -5) in component "ExPan"
extrude "Extrude35" add sketch "grid" along normal blind 1 separate body contours L0 L1 L2 L3 L8 L9 L10 L12 L13 L27 L29 | L2 L3 L7 L9 L11 L12 L27 L28 L30 | L3 L4 L5 L10 | L3 L4 L5 L11 | L3 L7 L25 L26 | L3 L13 L25 L26 | L3 L10 L17 L18 | L3 L11 L17 L18 | L3 L7 L23 L24 | L3 L13 L23 L24 | L3 L10 L19 L20 | L3 L11 L19 L20 | L3 L11 L21 L22 | L3 L10 L21 L22 | L3 L44 L45 L47 | L3 L43 L44 L45 | L3 L41 L42 L47 | L3 L41 L42 L43 | L3 L39 L40 L48 | L3 L32 L39 L40 | L3 L33 L34 L48 | L3 L32 L33 L34 | L3 L35 L36 L48 | L3 L32 L35 L36 | L3 L37 L38 L48 | L3 L32 L37 L38 | L15 L16 L51 L53 makes body 15 in component "ExPan"
extrude "Extrude34" [suppressed] in component "ExPan"
extrude "Extrude32" [suppressed] in component "ExPan"
component "ExPan" placed x (1, 0, 0) y (0, 1, 0) z (0, 0, 1) at (0, 0, 0)
hidden bodies 15
equation "d76 = pin_height"
equation "pin_height = 20 mm"
equation "pcb_height = 2 mm"
equation "base_height = 2 mm"
equation "mask_height = 1 mm"
equation "cell_height = 0.4 mm"
equation "d85 = base_height"
equation "pressa_height = 6 mm"
equation "d100 = 7 mm + 4.3 mm"
equation "d104 = 2.5 mm + 7 mm"
equation "d135 = base_height + 10 mm"
equation "d137 = base_height + 1 mm"
equation "d238 = cell_height"
equation "d244 = mask_height"
equation "d246 = pressa_height"
equation "d255 = pcb_height"
equation "d257 = cell_height"
equation "griglia_height = 1 mm"
equation "d276 = griglia_height"
equation "d330 = griglia_height"
equation "d368 = griglia_height"
named bodies: "Pin1", "Pin2", "Pin3", "Pin4", "Base", "cell1", "Mask", "Press", "PCB", "cell2", "grid"
